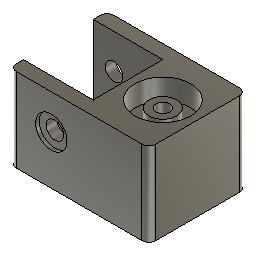
Bed Mount (Autodesk Fusion 360 design; units mm, degrees)
part number: Mount
Autodesk Fusion 360 part; units mm, degrees
sketch "Sketch1" plane through (0, 0, 0) normal (0, 0, 1) x (1, 0, 0) in component "Mount"
  line L0 (20, 14) -> (-20, 14)
  line L1 (-20, 14) -> (-20, -14)
  line L2 (-20, -14) -> (20, -14)
  line L3 (20, -14) -> (20, 14)
  line L4 (20, 14) -> (-20, -14) construction
  line L5 (-20, 14) -> (20, -14) construction
  dimension "d1" = 40
  dimension "d2" = 28
  constraint perpendicular L0 L1
  constraint parallel L0 L2
  constraint parallel L1 L3
  constraint horizontal L0
  constraint coincident L4 origin
  constraint coincident L5 origin
  measures "d1" distance of L1.end L2.end
  measures "d2" distance of L0.end L1.end
extrude "Extrude1" add sketch "Sketch1" along normal blind 24 in component "Mount"
sketch "Sketch2" plane through (0, 0, 24) normal (0, 0, 1) x (-1, 0, 0) in component "Mount"
  line L0 (-20, 14) -> (-20, -14)
  line L1 (-20, -14) -> (20, -14)
  line L2 (20, -14) -> (20, 14)
  line L3 (20, 14) -> (-20, 14)
  line L4 (20, -10) -> (0, -10)
  line L5 (0, -10) -> (0, 10)
  line L6 (0, 10) -> (20, 10)
  line L7 (20, 10) -> (20, -10)
  dimension "d5" = 20
  dimension "d6" = 20
  dimension "d7" = 4
  constraint horizontal L4
  constraint vertical L5
  constraint horizontal L6
  constraint vertical L7
  constraint coincident L2 L4.start
  measures "d5" distance of L4.start L6.end
  measures "d6" distance of L4.start L4.end
  measures "d7" distance of L1 L4
extrude "Extrude2" cut sketch "Sketch2" against normal blind 20 contours L2 L4 L5 L6 L7 in component "Mount"
sketch "Sketch3" plane through (0, -14, 0) normal (0, -1, 0) x (1, 0, 0) in component "Mount"
  line L0 (-20, 0) -> (20, 0)
  line L1 (20, 0) -> (20, 24)
  line L2 (20, 24) -> (-20, 24)
  line L3 (-20, 24) -> (-20, 0)
  line L4 (-8, 0) -> (-8, 24) construction
  line L5 (-20, 14) -> (20, 14) construction
  circle A0 centre (-8, 14) radius 2.5
  circle A1 centre (-8, 14) radius 4.5
  dimension "d10" = 12
  dimension "d11" = 10
  dimension "d12" = 5
  dimension "d13" = 9
  constraint coincident L0 L4.start
  constraint coincident L2 L4.end
  constraint perpendicular L2 L4
  constraint coincident L3 L5.start
  constraint coincident L1 L5.end
  constraint perpendicular L1 L5
  constraint coincident L5 A0.centre
  constraint coincident L4 A0.centre
  constraint concentric A0 A1
  measures "d10" distance of L3 L4
  measures "d11" distance of L2 L5
  measures "d12" diameter of A0
  measures "d13" diameter of A1
extrude "Extrude4" cut sketch "Sketch3" against normal blind 1 contours A0 | A1 in component "Mount"
extrude "Extrude3" cut sketch "Sketch3" against normal blind 4 contours A0 in component "Mount"
sketch "Sketch4" plane through (0, 14, 0) normal (0, 1, 0) x (-1, 0, 0) in component "Mount"
  line L0 (-20, 0) -> (20, 0)
  line L1 (20, 0) -> (20, 24)
  line L2 (20, 24) -> (-20, 24)
  line L3 (-20, 24) -> (-20, 0)
  line L4 (14, 24) -> (14, 0) construction
  line L5 (20, 14) -> (-20, 14) construction
  circle A0 centre (14, 14) radius 2.5
  circle A1 centre (14, 14) radius 4.5
  dimension "d18" = 10
  dimension "d19" = 6
  dimension "d20" = 5
  dimension "d21" = 9
  constraint coincident L2 L4.start
  constraint coincident L0 L4.end
  constraint perpendicular L0 L4
  constraint coincident L1 L5.start
  constraint coincident L3 L5.end
  constraint perpendicular L3 L5
  constraint coincident L5 A0.centre
  constraint coincident L4 A0.centre
  constraint concentric A0 A1
  measures "d18" distance of L2 L5
  measures "d19" distance of L1 L4
  measures "d20" diameter of A0
  measures "d21" diameter of A1
extrude "Extrude6" cut sketch "Sketch4" against normal blind 1 contours A0 | A1 in component "Mount"
extrude "Extrude5" cut sketch "Sketch4" against normal blind 4 contours A0 in component "Mount"
sketch "Sketch5" plane through (0, 0, 24) normal (0, 0, 1) x (-1, 0, 0) in component "Mount"
  line L0 (0, 10) -> (20, 10)
  line L1 (20, 10) -> (20, 14)
  line L2 (20, 14) -> (-20, 14)
  line L3 (-20, 14) -> (-20, -14)
  line L4 (-20, -14) -> (20, -14)
  line L5 (20, -14) -> (20, -10)
  line L6 (20, -10) -> (0, -10)
  line L7 (0, -10) -> (0, 10)
  line L8 (0, -10) -> (-20, -10) construction
  line L9 (0, 10) -> (-20, 10) construction
  line L10 (-20, 10) -> (0, -10) construction
  line L11 (0, 10) -> (-20, -10) construction
  circle A0 centre (-10, 0) radius 8
  circle A1 centre (-10, 0) radius 4
  circle A2 centre (-10, 0) radius 2
  dimension "d26" = 16
  dimension "d27" = 8
  dimension "d28" = 4
  constraint coincident L6.end L7.start
  constraint coincident L3 L8.end
  constraint perpendicular L3 L8
  constraint coincident L0.start L7.end
  constraint coincident L3 L9.end
  constraint perpendicular L3 L9
  constraint midpoint L11 A0.centre
  constraint concentric A0 A1
  constraint concentric A0 A2
  measures "d26" diameter of A0
  measures "d27" diameter of A1
  measures "d28" diameter of A2
extrude "Extrude7" cut sketch "Sketch5" against normal blind 6 contours A0 | A1 | A2 in component "Mount"
extrude "Extrude8" add sketch "Sketch5" along normal blind 4 from surface at -6 contours A1 in component "Mount"
extrude "Extrude9" cut sketch "Sketch5" against normal blind 18.3 contours A2 in component "Mount"
fillet "Fillet2" radius 2 4 edges at (20, 14, 12) (20, -14, 12) (-20, -14, 12) (-20, 14, 12) in component "Mount"
sketch "Sketch6" plane through (0, 0, 0) normal (0, 0, -1) x (1, 0, 0) in component "Mount"
  arc A0 (-20, -12) -> (-18, -14) centre (-18, -12) ccw
  line L0 (-18, -14) -> (18, -14)
  arc A1 (18, -14) -> (20, -12) centre (18, -12) ccw
  line L1 (20, -12) -> (20, 12)
  arc A2 (20, 12) -> (18, 14) centre (18, 12) ccw
  line L2 (18, 14) -> (-18, 14)
  arc A3 (-18, 14) -> (-20, 12) centre (-18, 12) ccw
  line L3 (-20, 12) -> (-20, -12)
  line L4 (12.8, -1.6166) -> (12.8, 1.6166)
  line L5 (12.8, 1.6166) -> (10, 3.2332)
  line L6 (10, 3.2332) -> (7.2, 1.6166)
  line L7 (7.2, 1.6166) -> (7.2, -1.6166)
  line L8 (7.2, -1.6166) -> (10, -3.2332)
  line L9 (10, -3.2332) -> (12.8, -1.6166)
  line L10 (10, 0) -> (10, 14) construction
  point P0 (10, 0)
  dimension "d50" = 2.8
  constraint coincident P0 L10.start
  constraint coincident L2 L10.end
  constraint perpendicular L2 L10
  constraint coincident L5.end L10
  measures "d50" distance of P0 L9
extrude "Extrude10" cut sketch "Sketch6" against normal blind 5.5 contours L4 L5 L6 L7 L8 L9 in component "Mount"
component "Mount" placed x (1, 0, 0) y (0, 1, 0) z (0, 0, 1) at (0, 0, 0)
